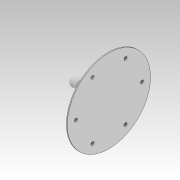
# Autodesk Inventor part: TrainingTarget
Saved by Autodesk Inventor 2020 (Build 240168000, 168)
## iProperties
Created: 2022-08-28
Part Number: TrainingTarget
Material: Generic
Document SubType Name: Modeling
Designer: DDeGo
Density: 1 g/cm^3
Appearance: Default
Author: DDeGo
Autodesk Inventor part; units mm, degrees
ref_plane "YZ Plane" through (0, 0, 0) normal (1, 0, 0) x (0, 1, 0)
ref_plane "XZ Plane" through (0, 0, 0) normal (0, 1, 0) x (-1, 0, 0)
sketch "Sketch1" plane through (0, 0, 0) normal (0, 0, 1) x (1, 0, 0)
  line L0 (0, 0) -> (0, 44)
  line L1 (-14.0215, 3) -> (-31, 3)
  arc A0 (-31, 3) -> (-40, 0) centre (-35, 0) ccw
  line L2 (-40, 0) -> (0, 0)
  line L3 (0, 44) -> (-1, 44)
  line L4 (-1, 44) -> (-9.1378, 6.928)
  arc A1 (-14.0215, 3) -> (-9.1378, 6.928) centre (-14.0215, 8) ccw
  point P0 (-10, 3)
  dimension "d0" = 44
  dimension "d1" = 5
  dimension "d2" = 3
  dimension "d3" = 1
  dimension "d4" = 35
  dimension "d5" = 10
  dimension "d18" = 5
  constraints: 10 end point, 4 point on circle, 3 point on line, 2 centre point, 2 horizontal, 2 tangent, 1 perpendicular, 1 vertical
  measures "d0" distance of L0.start L0.end
  measures "d1" radius of A0
  measures "d2" distance between parallel lines of L2 L1
  measures "d3" distance of L0.end L3.end
  measures "d4" distance from line of L0 A0.centre
  measures "d5" distance from line of L0 point (-10, 3)
  measures "d18" radius of A1
revolve "Revolution1" add sketch "Sketch1" angle 360 about axis through (-40, 0, 0) along (1, 0, 0)
sketch "Sketch2" plane through (0, 0, 0) normal (1, 0, 0) x (0, 0, -1)
  line L0 (0, 0) -> (35, 0) construction
  circle A0 centre (35, 0) radius 1.65
  dimension "d7" = 3.3
  dimension "d8" = 35
  constraints: 2 end point, 1 centre point, 1 coincident, 1 horizontal
  measures "d7" diameter of A0
  measures "d8" distance of L0.start L0.end
extrude "Extrusion1" cut sketch "Sketch2" against normal through all
ref_plane "Work Plane1" through (-2, 0, 0) normal (1, 0, 0) x (0, 0, -1)
sketch "Sketch3" plane through (-2, 0, 0) normal (1, 0, 0) x (0, 0, -1)
  circle A0 centre (35, 0) radius 3
  circle A1 centre (35, 0) radius 1.65 projected
  point P0 (0, 0)
  dimension "d12" = 6
  constraints: 1 centre point, 1 concentric
  measures "d12" diameter of A0
extrude "Extrusion2" cut sketch "Sketch3" against normal through all contours A0 | A1
pattern_circular "Circular Pattern1" count 6 over 360 about axis through (-22.5107, 0, 0) along (1, 0, 0) of "Extrusion2", "Extrusion1"
body "Solid1"
